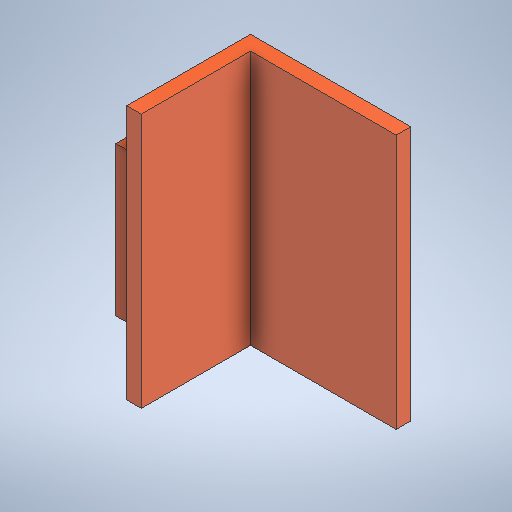
# Autodesk Inventor part: TapaTrasera
Saved by Autodesk Inventor 2025.1 (Build 291241020, 241B)
## iProperties
Created: 2024-08-31
Part Number: TapaTrasera
Material: Generic
Document SubType Name: Modeling
Designer: andre
Density: 1 g/cm^3
Appearance: Default
Author: andre
Autodesk Inventor part; units mm, degrees
ref_plane "YZ Plane" through (0, 0, 0) normal (1, 0, 0) x (0, 1, 0)
ref_plane "XZ Plane" through (0, 0, 0) normal (0, 1, 0) x (-1, 0, 0)
ref_plane "XY Plane" through (0, 0, 0) normal (0, 0, 1) x (1, 0, 0)
sketch "Sketch1" plane through (0, 0, 0) normal (0, 0, 1) x (1, 0, 0)
  line L0 (0, 0) -> (22, 0)
  line L1 (22, 0) -> (22, 35)
  line L2 (22, 35) -> (0, 35)
  line L3 (0, 35) -> (0, 0)
  dimension "d0" = 22
  dimension "d1" = 35
  constraints: 8 end point, 2 parallel, 1 horizontal, 1 perpendicular
  measures "d0" distance of L2.end L1.end
  measures "d1" distance of L1.end L0.end
extrude "Extrusion1" add sketch "Sketch1" along normal blind 2
sketch "Sketch2" plane through (0, 0, 2) normal (0, 0, 1) x (1, 0, 0)
  line L0 (0, 35) -> (0, 0) projected
  line L1 (0, 0) -> (2, 0)
  line L2 (2, 0) -> (2, 35)
  line L3 (2, 35) -> (0, 35)
  line L4 (0, 35) -> (0, 0)
  dimension "d4" = 2
  constraints: 8 end point, 2 parallel, 1 horizontal, 1 perpendicular
  measures "d4" distance between parallel lines of L0 L2
extrude "Extrusion2" add sketch "Sketch2" along normal blind 15
sketch "Sketch3" plane through (0, 0, 0) normal (-1, 0, 0) x (0, 0, 1)
  line L0 (15, 27.75) -> (8, 27.75)
  line L1 (8, 7.25) -> (15, 7.25)
  line L2 (15, 7.25) -> (15, 27.75)
  line L3 (8, 24.75) -> (6, 24.75)
  line L4 (6, 24.75) -> (6, 10.25)
  line L5 (6, 10.25) -> (8, 10.25)
  line L6 (8, 27.75) -> (8, 24.75)
  line L7 (8, 10.25) -> (8, 7.25)
  line L8 (17, 35) -> (17, 0) projected
  point P0 (0, 0)
  point P1 (17, 17.5)
  point P2 (15, 17.5)
  dimension "d7" = 20.5
  dimension "d8" = 2
  dimension "d9" = 7
  dimension "d10" = 2
  dimension "d11" = 14.5
  constraints: 16 end point, 4 parallel, 3 perpendicular, 2 horizontal, 2 midpoint, 1 collinear, 1 horizontal alignment, 1 vertical alignment
  measures "d7" distance of L1.end L0.start
  measures "d8" distance between parallel lines of L8 L2
  measures "d9" distance of L0.start L0.end
  measures "d10" distance between parallel lines of L6 L4
  measures "d11" distance of L3.end L4.end
extrude "Extrusion3" add sketch "Sketch3" along normal blind 3.5
equation "\"d2\" = w"
equation "\"d4\" = w"
equation "\"w\" = 2"
body "Solid1"
